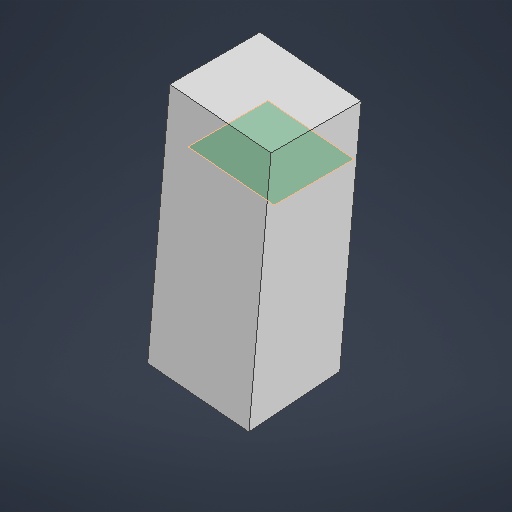
# Autodesk Inventor part: Part16
Saved by Autodesk Inventor 2026.2 (Build 302298010, 298A)
## iProperties
Created: 2026-05-20
Part Number: Part16
Material: Generic
Document SubType Name: Modeling
Designer: lenovo
Density: 1 g/cm^3
Appearance: Default
Author: lenovo
Autodesk Inventor part; units mm, degrees
ref_plane "YZ Plane" through (0, 0, 0) normal (1, 0, 0) x (0, 1, 0)
ref_plane "XY Plane" through (0, 0, 0) normal (0, 0, 1) x (1, 0, 0)
ref_plane "Work Plane1" through (0, 0, 0) normal (-0.0871557, -0.9961947, 0) x (0, 0, 1)
sketch "Sketch1" plane through (0, 0, 0) normal (-0.0871557, -0.9961947, 0) x (0, 0, 1)
  line L0 (0, 0) -> (-24.8884, 0)
  line L1 (-24.8884, 0) -> (-24.8884, 28.0603)
  line L2 (-24.8884, 28.0603) -> (0, 28.0603)
  line L3 (0, 28.0603) -> (0, 0)
  constraints: 8 end point, 2 parallel, 1 horizontal, 1 perpendicular
extrude "Extrusion1" add sketch "Sketch1" along normal blind 70
sketch "Sketch2" plane through (0, 0, -24.8884) normal (0.9961947, -0.0871557, 0) x (0, 0, 1)
  line L0 (24.8884, 70) -> (0, 70) projected
  line L1 (24.8884, 70) -> (0, 67.8226)
  line L2 (0, 0) -> (0, 70) projected
  line L3 (24.8884, 70) -> (49.8718, 70) construction
  line L4 (0, 67.8226) -> (0, 70)
  line L5 (0, 70) -> (24.8884, 70)
  point P0 (24.8884, 0)
  dimension "d3" = 175
  constraints: 8 end point, 1 equal length, 1 horizontal, 1 perpendicular, 1 point on line
  measures "d3" angle of L1 L3
extrude "Extrusion2" cut sketch "Sketch2" against normal through all
body "Solid1"
